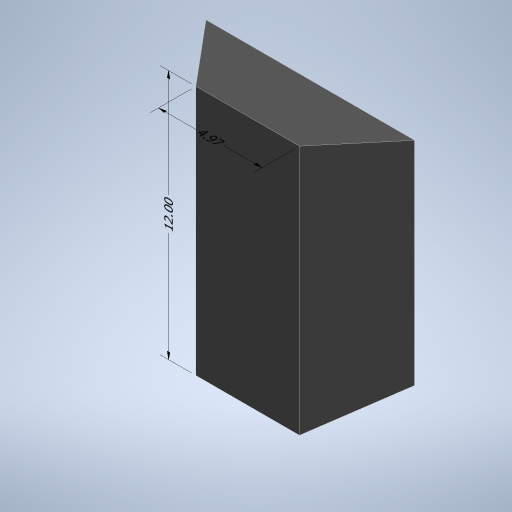
# Autodesk Inventor part: antana_middle
Saved by Autodesk Inventor 2024.1 (Build 281209000, 209)
## iProperties
Created: 2024-02-25
Part Number: antana_middle
Material: 一般
Document SubType Name: Modeling
Designer: hibik
Density: 1 g/cm^3
Appearance: 既定
Author: hibik
Autodesk Inventor part; units mm, degrees
ref_plane "YZ Plane" through (0, 0, 0) normal (1, 0, 0) x (0, 1, 0)
ref_plane "XZ Plane" through (0, 0, 0) normal (0, 1, 0) x (-1, 0, 0)
ref_plane "XY Plane" through (0, 0, 0) normal (0, 0, 1) x (1, 0, 0)
sketch "スケッチ1" plane through (0, 0, 0) normal (0, 0, 1) x (1, 0, 0)
  line L0 (-5, 12) -> (5, 12)
  line L1 (5, 12) -> (5, 0)
  line L2 (5, 0) -> (-5, 0)
  line L3 (-5, 0) -> (-5, 12)
  line L4 (-8.0749, 12) -> (-5, 12) construction
  point P0 (0, 0)
  point P1 (0, 12)
  point P2 (0, 0)
  dimension "d0" = 12
  dimension "d1" = 10
  dimension "d2" = 10
  constraints: 10 end point, 3 midpoint, 2 vertical alignment, 1 horizontal, 1 parallel, 1 perpendicular
  measures "d0" distance from line of L2.end L4
  measures "d1" distance of L0.start L0.end
  measures "d2" distance of L1.end L2.end
extrude "押し出し1" add sketch "スケッチ1" along normal blind 3
sketch "スケッチ2" plane through (-5, 12, 0) normal (0, 1, 0) x (1, 0, 0)
  line L0 (0, -3) -> (10, -3) projected
  line L1 (0, 0) -> (10, 0) projected
  line L2 (2.5173, -3) -> (0, 0)
  line L3 (10, 0) -> (7.4827, -3)
  line L4 (0, 0) -> (0, -3) projected
  line L5 (10, 0) -> (10, -3) projected
  point P0 (5, 0)
  dimension "d5" = 80
  dimension "d6" = 40
  dimension "d7" = 40
  constraints: 4 end point, 2 point on line
  measures "d5" angle of L3 L2
  measures "d6" angle of L4 L2
  measures "d7" angle of L5 L3
extrude "押し出し2" cut sketch "スケッチ2" against normal through all contours L4 L2 L0 | L3 L5 L0
sketch "スケッチ3" plane through (-5, 0, 0) normal (-0.7660444, 0, 0.6427876) x (0.6427876, 0, 0.7660444)
  line L0 (3.9162, 0) -> (0, 0) projected
  line L1 (3.9162, 12) -> (3.9162, 0) projected
  line L2 (0, 12) -> (3.9162, 12) projected
  line L3 (0, 12) -> (0, 0) projected
  line L4 (3.9162, 0) -> (7.1079, 0) projected
  line L5 (3.9162, 0) -> (-11.0838, 7)
  point P0 (3.2139, 0)
  point P1 (0, 1.8276)
  dimension "d10" = 15
  dimension "d11" = 7
  constraints: 2 end point
  measures "d10" distance from line of L1 L5.end
  measures "d11" distance from line of L0 L5.end
extrude "押し出し3" cut sketch "スケッチ3" against normal through all contours L0 L3 L5
sketch "スケッチ4" plane through (5, 0, 0) normal (0.7660444, 0, 0.6427876) x (0.6427876, 0, -0.7660444)
  line L0 (0, 0) -> (-3.9162, 0) projected
  line L1 (0, 0) -> (0, 12) projected
  line L2 (-3.9162, 12) -> (0, 12) projected
  line L3 (-3.9162, 0) -> (-3.9162, 12) projected
  line L4 (-3.9162, 0) -> (11.0838, 7)
  point P0 (-3.2139, 0)
  point P1 (0, 1.8276)
  dimension "d14" = 15
  dimension "d15" = 7
  constraints: 2 end point
  measures "d14" distance from line of L3 L4.end
  measures "d15" distance from line of L0 L4.end
extrude "押し出し4" cut sketch "スケッチ4" against normal through all contours L0 L4 L1
equation "\"d6\" = d7"
